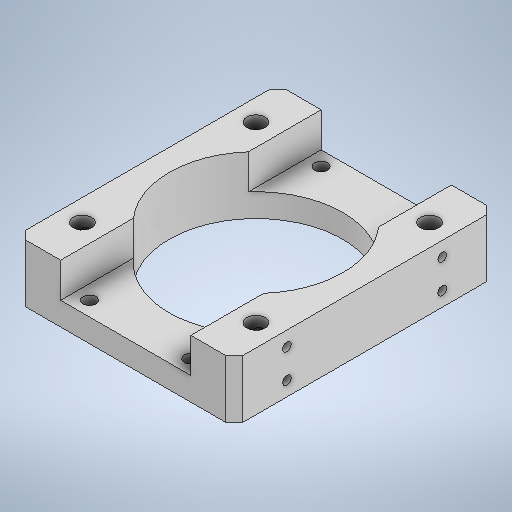
# Autodesk Inventor part: vertical_mount
Saved by Autodesk Inventor 2025.1 (Build 291241000, 241)
## iProperties
Created: 2024-12-03
Part Number: vertical_mount
Material: Ogólny
Document SubType Name: Modeling
Designer: PC
Density: 1 g/cm^3
Appearance: Domyślna
Author: PC
Autodesk Inventor part; units mm, degrees
ref_plane "YZ Plane" through (0, 0, 0) normal (1, 0, 0) x (0, 1, 0)
ref_plane "XZ Plane" through (0, 0, 0) normal (0, 1, 0) x (-1, 0, 0)
ref_plane "XY Plane" through (0, 0, 0) normal (0, 0, 1) x (1, 0, 0)
sketch "Szkic1" plane through (0, 0, 0) normal (0, 1, 0) x (-1, 0, 0)
  line L0 (0, 0) -> (60, 0) construction
  line L1 (60, 0) -> (60, -60) construction
  line L2 (60, -60) -> (0, -60) construction
  line L3 (0, -60) -> (0, 0) construction
  circle A0 centre (60, -60) radius 3.175
  circle A1 centre (60, 0) radius 3.175
  circle A2 centre (0, 0) radius 3.175
  circle A3 centre (0, -60) radius 3.175
  line L4 (47.5, 10) -> (12.5, 10) construction
  line L5 (12.5, 10) -> (12.5, -70) construction
  line L6 (12.5, -70) -> (47.5, -70) construction
  line L7 (47.5, -70) -> (47.5, 10) construction
  line L8 (12.5, 10) -> (47.5, -70) construction
  line L9 (47.5, 10) -> (12.5, -70) construction
  circle A4 centre (47.5, 10) radius 2.25
  circle A5 centre (47.5, -70) radius 2.25
  circle A6 centre (12.5, -70) radius 2.25
  circle A7 centre (12.5, 10) radius 2.25
  line L10 (-7.5, 15) -> (67.5, 15)
  line L11 (67.5, 15) -> (67.5, -75)
  line L12 (67.5, -75) -> (-7.5, -75)
  line L13 (-7.5, -75) -> (-7.5, 15)
  circle A8 centre (30, -30) radius 30
  point P0 (30, -30)
  point P1 (30, -60)
  point P2 (60, -30)
  point P3 (30, 15)
  point P4 (30, 10)
  point P5 (67.5, -30)
  dimension "d0" = 60
  dimension "d1" = 60
  dimension "d2" = 6.35
  dimension "d3" = 35
  dimension "d4" = 80
  dimension "d5" = 4.5
  dimension "d6" = 90
  dimension "d7" = 75
  dimension "d10" = 60
  constraints: 28 end point, 9 centre point, 9 coincident, 7 midpoint, 6 equal radius, 6 parallel, 3 horizontal, 3 perpendicular, 2 horizontal alignment, 2 vertical alignment
  measures "d0" distance of L1.end L2.end
  measures "d1" distance of L0.end L1.end
  measures "d2" diameter of A0
  measures "d3" distance of L6.end L5.end
  measures "d4" distance of L5.end L4.end
  measures "d5" diameter of A4
  measures "d6" distance of L10.end L11.end
  measures "d7" distance between parallel lines of L13 L11
  measures "d10" diameter of A8
extrude "Wyciągnięcie proste1" add sketch "Szkic1" along normal blind 20
sketch "Szkic2" plane through (7.5, 0, 15) normal (1, 0, 0) x (0, 0, -1)
  line L0 (11.825, 20) -> (11.825, 0) projected
  line L1 (18.175, 20) -> (18.175, 0) projected
  circle A0 centre (18.175, 15) radius 1.5
  circle A1 centre (18.175, 5) radius 1.5
  line L2 (0, 20) -> (90, 20) projected
  line L3 (0, 0) -> (90, 0) projected
  line L4 (45, 20) -> (45, 0) construction
  line L5 (15, 0) -> (75, 0) construction
  circle A2 centre (71.825, 15) radius 1.5
  circle A3 centre (71.825, 5) radius 1.5
  dimension "d13" = 3
  dimension "d14" = 5
  dimension "d15" = 5
  constraints: 4 centre point, 2 end point, 2 midpoint, 2 point on line, 2 symmetric about line, 1 equal radius, 2 other
  measures "d13" diameter of A0
  measures "d14" distance from line of L2 A0.centre
  measures "d15" distance from line of L3 A1.centre
extrude "Wyciągnięcie proste2" cut sketch "Szkic2" against normal blind 12.25 contours A0 L1 | L1 A0 | A1 L1 | L1 A1 | A2 | A3
pattern_circular "Szyk kołowy1" count 2 over 360 about axis through (-30, 0, -30) along (0, 1, 0) of "Wyciągnięcie proste2"
chamfer "Faza1" distance 3 angle 45 4 edges at (7.5, 10, 15) (7.5, 10, -75) (-67.5, 10, -75) (-67.5, 10, 15)
sketch "Szkic3" plane through (0, 20, 0) normal (0, 1, 0) x (1, 0, 0)
  line L0 (4.5, 75) -> (-64.5, 75) projected
  line L1 (-64.5, -15) -> (4.5, -15) projected
  line L2 (-7.5, 75) -> (-52.5, 75)
  line L3 (-52.5, 75) -> (-52.5, -15)
  line L4 (-52.5, -15) -> (-7.5, -15)
  line L5 (-7.5, -15) -> (-7.5, 75)
  line L6 (-7.5, 75) -> (-52.5, -15) construction
  line L7 (-7.5, -15) -> (-52.5, 75) construction
  line L8 (7.5, -12) -> (7.5, 72) construction
  point P0 (0, 0)
  point P1 (-30, 30)
  point P2 (-30, -15)
  point P3 (-30, 30)
  point P4 (7.5, 30)
  point P5 (-7.5, -15)
  dimension "d24" = 45
  constraints: 12 end point, 4 midpoint, 2 parallel, 2 point on line, 1 horizontal, 1 horizontal alignment, 1 perpendicular, 1 vertical alignment
  measures "d24" distance between parallel lines of L3 L5
extrude "Wyciągnięcie proste3" cut sketch "Szkic3" against normal blind 12
sketch "Szkic4" plane through (0, 8, 0) normal (0, 1, 0) x (1, 0, 0)
  point P0 (0, 0)
